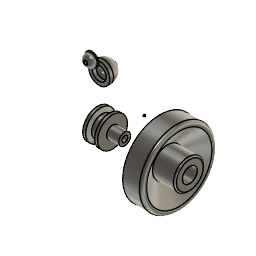
random components (Autodesk Fusion 360 design; units mm, degrees)
part number: 2026-04-16-20-34-28-016
part number: 2026-04-16-21-52-40-504
part number: 2026-04-16-21-52-47-722
part number: 2026-04-16-21-54-32-702
part number: 2026-04-16-21-56-28-893
Autodesk Fusion 360 part; units mm, degrees
note: some values were not read from the file. Set by a fixed rule: which sketch regions a step uses.
sketch "Sketch1" plane through (0, 0, 0) normal (0, 0, 1) x (1, 0, 0)
  line L0 (-200, 130) -> (-200, 50)
  line L1 (-200, 50) -> (-18.2042, 50)
  line L2 (-18.2042, 50) -> (-18.2042, 70)
  line L3 (-18.2042, 70) -> (-100, 70)
  line L4 (-100, 70) -> (-100, 130)
  line L5 (-100, 130) -> (-120, 130)
  line L6 (-120, 130) -> (-140, 100)
  line L7 (-140, 100) -> (-170, 100)
  line L8 (-170, 100) -> (-180, 130)
  line L9 (-180, 130) -> (-200, 130)
  line L10 (-250, 30) -> (0, 30)
  constraint vertical L0
  constraint perpendicular L0 L1
  constraint perpendicular L1 L2
  constraint perpendicular L0 L3
  constraint perpendicular L3 L4
  constraint perpendicular L0 L5
  constraint parallel L5 L7
  constraint perpendicular L0 L9
  constraint perpendicular L2 L10
revolve "Revolve1" add sketch "Sketch1" angle 360 about axis through (-250, 30, 0) along (1, 0, 0) makes body 1
sketch "Sketch2" plane through (0, 0, 0) normal (0, 0, 1) x (1, 0, 0)
  line L0 (100, 150) -> (100, -50)
  line L1 (100, -50) -> (300, -50)
  line L2 (300, -50) -> (300, -10)
  line L3 (290, 0) -> (150, 0)
  line L4 (150, 0) -> (229.2707, 118.906)
  line L5 (212.6297, 150) -> (100, 150)
  arc A0 (229.2707, 118.906) -> (212.6297, 150) centre (212.6297, 130) ccw
  arc A1 (300, -10) -> (290, 0) centre (290, -10) ccw
  line L6 (50, -100) -> (370, -100)
  dimension "d2" = 20
  dimension "d3" = 10
  constraint vertical L0
  constraint perpendicular L0 L1
  constraint perpendicular L1 L2
  constraint perpendicular L0 L3
  constraint perpendicular L0 L5
  constraint tangent L5 A0
  constraint tangent L4 A0
  constraint tangent L3 A1
  constraint tangent L2 A1
  constraint horizontal L6
  measures "d2" radius of A0
  measures "d3" radius of A1
revolve "Revolve2" add sketch "Sketch2" angle 360 about axis through (50, -100, 0) along (1, 0, 0) separate body makes body 2
copy_body "Body->Comp1" bodies 1 removing the originals makes body 3 in component "Component"
copy_body "Body->Comp2" bodies 2 removing the originals makes body 4 in component "Component'"
sketch "Sketch3" plane through (0, 0, 0) normal (0, 0, 1) x (1, 0, 0)
  line L0 (25, 250) -> (25, 200)
  arc A0 (25, 200) -> (50, 175) centre (50, 200) ccw
  line L1 (50, 175) -> (50, 150)
  line L2 (50, 150) -> (75, 150)
  line L3 (75, 150) -> (75, 175)
  arc A1 (75, 175) -> (25, 250) centre (-6.25, 175) ccw
  line L4 (3.8146, 256.3756) -> (3.8146, 150)
  constraint vertical L0
  constraint tangent L0 A0
  constraint parallel L0 L1
  constraint perpendicular L1 L2
  constraint perpendicular L2 L3
  constraint tangent L3 A1
  constraint parallel L0 L4
revolve "Revolve3" add sketch "Sketch3" angle 360 about axis through (3.8146, 256.3756, 0) along (0, -1, 0) separate body makes body 5
copy_body "Body->Comp3" bodies 5 removing the originals makes body 6 in component "Component''"
sketch "Sketch4" plane through (0, 0, 0) normal (0, 0, 1) x (1, 0, 0)
  line L0 (-150, 240) -> (-150, 213)
  arc A0 (-154, 195) -> (-150, 213) centre (-192.5, 213) ccw
  line L1 (-154, 195) -> (-150, 195)
  arc A1 (-150, 195) -> (-123, 231) centre (-150, 223.125) ccw
  arc A2 (-118, 237) -> (-123, 231) centre (-118.4815, 232.3179) ccw
  line L2 (-118, 237) -> (-123, 241)
  arc A3 (-115, 243) -> (-123, 241) centre (-119.7619, 245.0476) ccw
  line L3 (-115, 243) -> (-150, 240)
  line L4 (-164.2022, 250.0763) -> (-164.2022, 180)
  constraint vertical L0
  constraint tangent L0 A0
  constraint perpendicular L0 L1
  constraint tangent L1 A1
  constraint tangent A1 A2
  constraint tangent L2 A3
  constraint parallel L0 L4
revolve "Revolve4" add sketch "Sketch4" angle 360 about axis through (-164.2022, 250.0763, 0) along (0, -1, 0) separate body contours L0 A0 L1 A1 A2 L2 A3 L3 makes body 7
copy_body "Body->Comp4" bodies 7 removing the originals makes body 8 in component "Component'''"
sketch "Sketch5" plane through (0, 0, 0) normal (0, 0, 1) x (1, 0, 0)
  line L0 (-200.6341, 95.1359) -> (-200.6341, 70.2872)
  arc A0 (-201.118, 91.4572) -> (-200.1501, 91.4572) centre (-200.6341, 93.4321) ccw
  arc A1 (-200.1501, 91.4572) -> (-200.6341, 86.0339) centre (-200.6341, 88.7671) ccw
  arc A2 (-200.6341, 86.0158) -> (-200.6341, 79.8162) centre (-200.6341, 82.916) ccw
  arc A3 (-200.6341, 79.7128) -> (-200.6341, 70.2872) centre (-200.6341, 75) ccw
  line L1 (-203, 97) -> (-161, 70)
  constraint vertical L0
  constraint coincident L0 A3.centre
  constraint coincident L0 A1.centre
  constraint coincident L0 A0.centre
  constraint coincident A0.start A1
  constraint coincident L0 A1.end
  constraint coincident L0 A2.end
  constraint coincident L0 A2.start
  constraint coincident L0 A2.centre
  constraint coincident L0 A3.start
revolve "Revolve5" add sketch "Sketch5" angle 360 about axis through (-203, 97, 0) along (0.841178, -0.540758, 0) separate body contours L0 A0 A1 picked at (-200.7686, 87.8322) makes body 9
component "Component" placed x (1, 0, 0) y (0, 1, 0) z (0, 0, 1) at (98.1737, -143.586, 49.6266)
component "Component'" placed x (1, 0, 0) y (0, 1, 0) z (0, 0, 1) at (0, 0, 0)
component "Component''" placed x (1, 0, 0) y (0, 1, 0) z (0, 0, 1) at (59.9723, 41.7499, -5.1853)
component "Component'''" placed x (1, 0, 0) y (0, 1, 0) z (0, 0, 1) at (132.3706, -161.9802, 104.6859)
